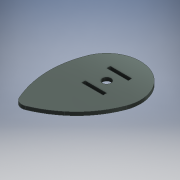
# Autodesk Inventor part: leva00
Saved by Autodesk Inventor 2016 (Build 200138000, 138)
## iProperties
Created: 2016-09-20
Part Number: leva00
Material: Madera (abedul)
Document SubType Name: Modeling
Designer: i95sa
Density: 0.55 g/cm^3
Appearance: Gris plomo - Pulido
Author: i95sa
Autodesk Inventor part; units mm, degrees
ref_plane "YZ Plane" through (0, 0, 0) normal (1, 0, 0) x (0, 1, 0)
ref_plane "XZ Plane" through (0, 0, 0) normal (0, 1, 0) x (-1, 0, 0)
ref_plane "XY Plane" through (0, 0, 0) normal (0, 0, 1) x (1, 0, 0)
sketch "Boceto1" plane through (0, 0, 0) normal (0, 0, 1) x (1, 0, 0)
  arc A0 (14.3808, 36.3217) -> (-14.3808, -36.3217) centre (0, 0) ccw
  arc A1 (-22.1309, -55.8963) -> (-28.7682, -72.6601) centre (-25.4495, -64.2782) ccw
  line L0 (-29.729, -75.0869) -> (-38.111, -71.7683)
  line L1 (-36.1488, 14.81) -> (-50.1187, 20.3411)
  line L2 (-50.1187, 20.3411) -> (-38.111, -71.7683)
  line L3 (-38.111, -71.7683) -> (-42.7724, -36.0108)
  arc A2 (-36.1488, 14.81) -> (-42.7724, -36.0108) centre (56.3545, -23.0882) ccw
  arc A3 (-42.7724, -36.0108) -> (-33.6613, -67.9981) centre (69.1643, -21.4183) ccw
  line L4 (1.1062, 2.794) -> (14.3808, 36.3217)
  line L5 (-1.1062, -2.794) -> (-29.729, -75.0869)
  arc A4 (-14.3808, -36.3217) -> (14.3808, 36.3217) centre (0, 0) ccw
  arc A5 (-28.7682, -72.6601) -> (-22.1309, -55.8963) centre (-25.4495, -64.2782) ccw
  line L6 (-29.729, -75.0869) -> (-21.3471, -78.4056)
  line L7 (36.4895, -13.9495) -> (50.4594, -19.4806)
  line L8 (50.4594, -19.4806) -> (-21.3471, -78.4056)
  line L9 (-21.3471, -78.4056) -> (6.5286, -55.5305)
  arc A6 (6.5286, -55.5305) -> (36.4895, -13.9495) centre (-56.8857, 21.7467) ccw
  arc A7 (-22.0099, -72.6112) -> (6.5286, -55.5305) centre (-65.0805, 31.733) ccw
  dimension "d0" = 78.13
  dimension "d6" = 18.03
  dimension "d7" = 9.015
  dimension "d8" = 15.025
  dimension "d9" = 36.06
  constraints: 20 end point, 20 point on circle, 8 centre point, 6 symmetric about line, 5 point on line, 4 tangent, 1 collinear, 4 other
  measures "d0" diameter of A0
  measures "d6" diameter of A1
  measures "d7" distance of L0.start L0.end
  measures "d8" distance of L1.start L1.end
  measures "d9" distance of L0.end L3.end
extrude "Extrusión2" add sketch "Boceto1" along normal blind 4 contours A4 A0 | A0 L5 A1 A3 A2 | A6 A7 A5 L5 A4 | L5 A1 | A5 L5
sketch "Boceto2" plane through (0, 0, 4) normal (0, 0, 1) x (1, 0, 0)
  line L0 (0, 0) -> (0, 12.5)
  line L1 (0, 12.5) -> (-12.5, 12.5)
  line L2 (-12.5, 12.5) -> (-12.5, 16.7)
  line L3 (-12.5, 16.7) -> (12.5, 16.7)
  line L4 (12.5, 16.7) -> (12.5, 12.5)
  line L5 (12.5, 12.5) -> (0, 12.5)
  line L6 (0, 0) -> (12.5, 0)
  line L7 (0, 0) -> (0, -12.5)
  line L8 (0, -12.5) -> (-12.5, -12.5)
  line L9 (-12.5, -12.5) -> (-12.5, -16.7)
  line L10 (-12.5, -16.7) -> (12.5, -16.7)
  line L11 (12.5, -16.7) -> (12.5, -12.5)
  line L12 (12.5, -12.5) -> (0, -12.5)
  circle A0 centre (0, 0) radius 5
  dimension "d24" = 12.5
  dimension "d25" = 12.5
  dimension "d26" = 4.2
  dimension "d27" = 25
  dimension "d28" = 10
  constraints: 26 end point, 5 perpendicular, 5 symmetric about line, 3 point on line, 1 centre point, 1 coincident, 1 parallel, 1 vertical
  measures "d24" distance of L0.start L0.end
  measures "d25" distance of L0.end L1.end
  measures "d26" distance of L1.end L2.end
  measures "d27" distance of L2.end L3.end
  measures "d28" diameter of A0
extrude "Extrusión3" cut sketch "Boceto2" against normal blind 4
